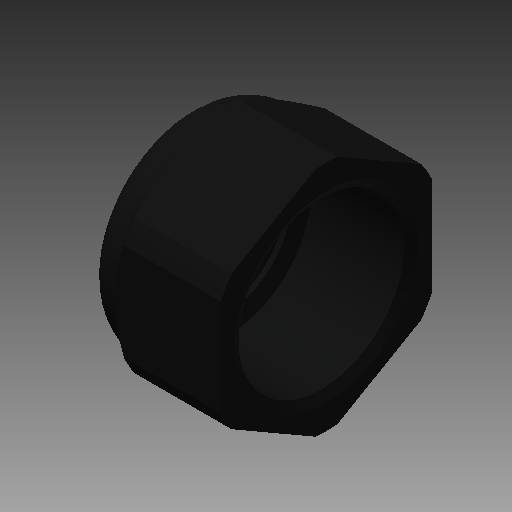
# Autodesk Inventor part: HSK-K 1.209.1201.70-Nut
Saved by Autodesk Inventor 2018 (Build 220112000, 112)
## iProperties
Category: PARTsolutions
Company: SEALCON
Created: 2018-02-18
Part Number: HSK-K 1.209.1201.70-Nut
Catalog Web Link: www.cadenas.de
Description: HSK-K NPT-Nut-Industrial cable glands
Vendor: SEALCON
Document SubType Name: Modeling
Designer: psAdmin
Manufacturer: SEALCON
Mass: 3.72932 g
Surface Area: 26.4903 cm^2
Volume: 3.72932 cm^3
Density: 1 g/cm^3
Material: Generic
Appearance: PSOLRGB-10-10-10
PSOL_IDENT_0: {$CADENAS_DATA\23d-libs\sealcon\kabelverschraubungen\industriekabelverschraubungen\hsk_standard_kabe
PSOL_IDENT_1: lver\hsk_k\npt\hsk_k_npt_nut.prj},209 {VTYP=3D},{NB=HSK-K 1.209.1201.70-Nut},{LINA=HSK-K 1.209.1201.
PSOL_IDENT_2: 70-Nut},{NN=HSK-K NPT-Nut},{DATE=25.01.2018 07:57:44},{GEOMDATE=03.03.2011 00:00:00},{VERSION=v11071
PSOL_IDENT_3: 8060127},{LINEID=200},{LINESUBID=-1},{WBVAR=}  {NB=HSK-K 1.209.1201.70_nut},{LINA=HSK-K 1.209.1201.7
PSOL_IDENT_4: 0_nut},{KT=DUMMY},{AG=1/2\" NPT},{FR=black},{GL=13},{H=27},{SW=24},{BN=1.209.1201.70},{COLX=0.04,0.0
PSOL_IDENT_5: 4,0.04,0.00},{VER=2}
NN: HSK-K NPT-Nut
NT: Industrial cable glands
NB: HSK-K 1.209.1201.70-Nut
NBSYN: HSK-K $BN.-Nut
LINA: HSK-K 1.209.1201.70-Nut
AG: 1/2" NPT
FR: black
GL: 13
H: 27
SW: 24
BN: 1.209.1201.70
VER: 2
SUPPLIER: SEALCON
ARTICLENO: HSK-K 1.209.1201.70-Nut
BOMINFO: HSK-K 1.209.1201.70-Nut
CREATOR: CADENAS GmbH
Title: HSK-K 1.209.1201.70-Nut
Author: Cadenas PARTsolutions
Comments: Industrial cable glands
Autodesk Inventor part; units mm, degrees
sketch "Sketch_1" plane through (0, 0, 0) normal (0, 0, 1) x (1, 0, 0)
  line L0 (16, 0) -> (0, 0)
  line L1 (0, 0) -> (0, 8.35)
  arc A0 (3.5, 11.85) -> (0, 8.35) centre (3.5, 8.35) ccw
  line L2 (3.5, 11.85) -> (3.6341, 11.85)
  arc A1 (3.6341, 11.85) -> (4.0171, 12.0286) centre (3.6341, 12.35) ccw
  line L3 (4.0171, 12.0286) -> (5, 13.2)
  line L4 (5, 13.2) -> (16, 13.2)
  line L5 (16, 13.2) -> (16, 0)
  line L6 (16, 0) -> (0, 0)
  constraints: 14 end point, 4 point on circle, 2 centre point
revolve "Revolution1" add sketch "Sketch_1" angle 360 about axis through (16, 0, 0) along (1, 0, 0)
sketch "Sketch_2" plane through (0, 0, 0) normal (1, 0, 0) x (0, 1, 0)
  line L0 (-24, 24) -> (-24, -24)
  line L1 (-24, -24) -> (24, -24)
  line L2 (24, -24) -> (24, 24)
  line L3 (24, 24) -> (-24, 24)
  line L4 (-6.9282, 12) -> (-13.8564, 0)
  line L5 (-13.8564, 0) -> (-6.9282, -12)
  line L6 (-6.9282, -12) -> (6.9282, -12)
  line L7 (6.9282, -12) -> (13.8564, 0)
  line L8 (13.8564, 0) -> (6.9282, 12)
  line L9 (6.9282, 12) -> (-6.9282, 12)
  constraints: 20 end point
extrude "Extrusion1" cut sketch "Sketch_2" along normal blind 16
sketch "Sketch_3" plane through (0, 0, 0) normal (0, 0, 1) x (1, 0, 0)
  line L0 (16, 0) -> (-0.2, 0)
  line L1 (-0.2, 0) -> (-0.2, 7.05)
  line L2 (-0.2, 7.05) -> (0, 7.05)
  arc A0 (0, 7.05) -> (1, 6.05) centre (1, 7.05) ccw
  line L3 (1, 6.05) -> (2.554, 6.05)
  arc A1 (2.554, 6.05) -> (3.7, 6.6458) centre (2.554, 7.45) ccw
  line L4 (3.7, 6.6458) -> (3.7, 7.85)
  line L5 (3.7, 7.85) -> (4.2447, 7.85)
  line L6 (4.2447, 7.85) -> (4.8414, 9.2557)
  arc A2 (4.8874, 9.35) -> (4.8414, 9.2557) centre (5.7619, 8.865) ccw
  line L7 (4.8874, 9.35) -> (6.8, 9.35)
  line L8 (6.8, 9.35) -> (6.8, 9.3)
  line L9 (6.8, 9.3) -> (15.419, 9.3937)
  line L10 (15.419, 9.3937) -> (16, 10.4)
  line L11 (16, 10.4) -> (16, 0)
  line L12 (16, 0) -> (-0.2, 0)
  constraints: 26 end point, 6 point on circle, 3 centre point
revolve "Revolution2" cut sketch "Sketch_3" angle 360 about axis through (16, 0, 0) along (1, 0, 0)
ref_plane "IP1_XY" through (0, 0, 0) normal (1, 0, 0) x (0, 0, -1)
ref_plane "IP1_YZ" through (0, 0, 0) normal (0, 0, -1) x (0, 1, 0)
ref_plane "IP1_ZX" through (0, 0, 0) normal (0, 1, 0) x (1, 0, 0)
body "Solid1"
